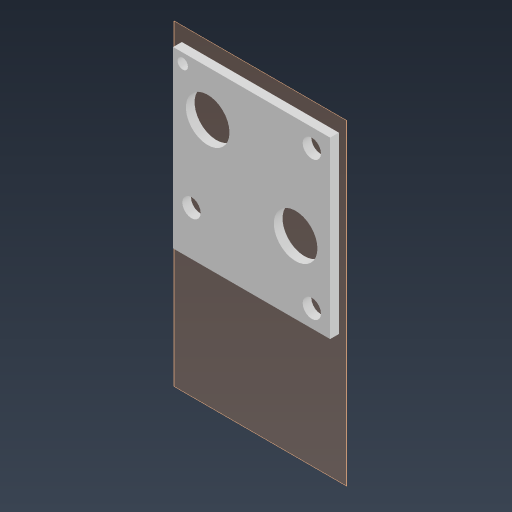
# Autodesk Inventor part: water line connector
Saved by Autodesk Inventor 2024.3 (Build 283343000, 343)
## iProperties
Created: 2024-03-20
Part Number: water line connector
Material: Generic
Document SubType Name: Modeling
Designer: mateu
Density: 1 g/cm^3
Appearance: Default
Author: mateu
Autodesk Inventor part; units mm, degrees
ref_plane "YZ Plane" through (0, 0, 0) normal (1, 0, 0) x (0, 1, 0)
ref_plane "XZ Plane" through (0, 0, 0) normal (0, 1, 0) x (-1, 0, 0)
ref_plane "Work Plane1" through (-8, -18, 2.25) normal (0, 0, 1) x (1, 0, 0)
ref_plane "Work Plane2" through (16.1776, -21.6969, -6.3588) normal (0, 0, 1) x (1, 0, 0)
sketch "Sketch6" plane through (16.1776, -21.6969, -6.3588) normal (0, 0, 1) x (1, 0, 0)
  circle A0 centre (6.9, -9.5) radius 1.2 projected
  circle A1 centre (-6.9, -6.4) radius 1.2 projected
  circle A2 centre (6.9, 6.4) radius 1.2 projected
  circle A3 centre (-7.9, 7.4) radius 0.4 projected
  line L0 (4.2, -7) -> (-1.2, -7) projected
  arc A4 (-8.5, 0.3) -> (-1.2, -7) centre (-1.2, 0.3) ccw projected
  line L1 (-8.5, 0.3) -> (-8.5, 2.7) projected
  arc A5 (-4.2, 7) -> (-8.5, 2.7) centre (-4.2, 2.7) ccw projected
  line L2 (-4.2, 7) -> (1.2, 7) projected
  arc A6 (8.5, -0.3) -> (1.2, 7) centre (1.2, -0.3) ccw projected
  line L3 (8.5, -0.3) -> (8.5, -2.7) projected
  arc A7 (4.2, -7) -> (8.5, -2.7) centre (4.2, -2.7) ccw projected
  line L4 (-4.2738, -7.5) -> (-4.2738, -24.5) projected
  line L5 (-4.2738, -7.5) -> (4.2738, -7.5) projected
  line L6 (4.2738, -24.5) -> (4.2738, -7.5) projected
  line L7 (9, -24.5) -> (4.2738, -24.5) projected
  line L8 (9, -24.5) -> (9, 8.5) projected
  line L9 (9, 8.5) -> (-9, 8.5) projected
  line L10 (-9, 8.5) -> (-9, -24.5) projected
  line L11 (-4.2738, -24.5) -> (-9, -24.5) projected
  line L12 (1.2, 6.2) -> (-4.2, 6.2) projected
  arc A8 (-4.2, 6.2) -> (-7.7, 2.7) centre (-4.2, 2.7) ccw projected
  line L13 (-7.7, 2.7) -> (-7.7, 0.3) projected
  arc A9 (-7.7, 0.3) -> (-1.2, -6.2) centre (-1.2, 0.3) ccw projected
  line L14 (-1.2, -6.2) -> (4.2, -6.2) projected
  arc A10 (4.2, -6.2) -> (7.7, -2.7) centre (4.2, -2.7) ccw projected
  line L15 (7.7, -2.7) -> (7.7, -0.3) projected
  arc A11 (7.7, -0.3) -> (1.2, 6.2) centre (1.2, -0.3) ccw projected
  line L16 (-7.2, 0.3) -> (-7.2, 2.7) projected
  arc A12 (-4.2, 5.7) -> (-7.2, 2.7) centre (-4.2, 2.7) ccw projected
  line L17 (-4.2, 5.7) -> (1.2, 5.7) projected
  arc A13 (7.2, -0.3) -> (1.2, 5.7) centre (1.2, -0.3) ccw projected
  line L18 (7.2, -0.3) -> (7.2, -2.7) projected
  arc A14 (4.2, -5.7) -> (7.2, -2.7) centre (4.2, -2.7) ccw projected
  line L19 (4.2, -5.7) -> (-1.2, -5.7) projected
  arc A15 (-7.2, 0.3) -> (-1.2, -5.7) centre (-1.2, 0.3) ccw projected
  line L20 (8.5, -0.3) -> (8.5, -2.7) projected
  arc A16 (8.5, -0.3) -> (1.2, 7) centre (1.2, -0.3) ccw projected
  line L21 (-4.2, 7) -> (1.2, 7) projected
  arc A17 (-4.2, 7) -> (-8.5, 2.7) centre (-4.2, 2.7) ccw projected
  line L22 (-8.5, 0.3) -> (-8.5, 2.7) projected
  arc A18 (-8.5, 0.3) -> (-1.2, -7) centre (-1.2, 0.3) ccw projected
  line L23 (4.2, -7) -> (-1.2, -7) projected
  arc A19 (4.2, -7) -> (8.5, -2.7) centre (4.2, -2.7) ccw projected
  arc A20 (-4.2, 6.2) -> (-7.7, 2.7) centre (-4.2, 2.7) ccw projected
  line L24 (1.2, 6.2) -> (-4.2, 6.2) projected
  arc A21 (7.7, -0.3) -> (1.2, 6.2) centre (1.2, -0.3) ccw projected
  line L25 (7.7, -2.7) -> (7.7, -0.3) projected
  arc A22 (4.2, -6.2) -> (7.7, -2.7) centre (4.2, -2.7) ccw projected
  line L26 (-1.2, -6.2) -> (4.2, -6.2) projected
  arc A23 (-7.7, 0.3) -> (-1.2, -6.2) centre (-1.2, 0.3) ccw projected
  line L27 (-7.7, 2.7) -> (-7.7, 0.3) projected
  line L28 (-1.4516, 1.7) -> (-0.5158, 1.7) projected
  arc A24 (2.07, 0.2211) -> (-0.5158, 1.7) centre (-0.5158, -1.3) ccw projected
  line L29 (2.07, 0.2211) -> (2.3135, -0.193) projected
  arc A25 (1.4516, -1.7) -> (2.3135, -0.193) centre (1.4516, -0.7) ccw projected
  line L30 (1.4516, -1.7) -> (0.5158, -1.7) projected
  arc A26 (-2.07, -0.2211) -> (0.5158, -1.7) centre (0.5158, 1.3) ccw projected
  line L31 (-2.07, -0.2211) -> (-2.3135, 0.193) projected
  arc A27 (-1.4516, 1.7) -> (-2.3135, 0.193) centre (-1.4516, 0.7) ccw projected
  arc A28 (-7.2, 0.3) -> (-1.2, -5.7) centre (-1.2, 0.3) ccw projected
  line L32 (-1.2, -5.7) -> (4.2, -5.7) projected
  arc A29 (4.2, -5.7) -> (7.2, -2.7) centre (4.2, -2.7) ccw projected
  line L33 (7.2, -2.7) -> (7.2, -0.3) projected
  arc A30 (7.2, -0.3) -> (1.2, 5.7) centre (1.2, -0.3) ccw projected
  line L34 (1.2, 5.7) -> (-4.2, 5.7) projected
  arc A31 (-4.2, 5.7) -> (-7.2, 2.7) centre (-4.2, 2.7) ccw projected
  line L35 (-7.2, 2.7) -> (-7.2, 0.3) projected
  line L36 (-9, 8.5) -> (9, 8.5)
  line L37 (9, 8.5) -> (9, -11.5)
  line L38 (9, -11.5) -> (-9, -11.5)
  line L39 (-9, -11.5) -> (-9, 8.5)
  circle A32 centre (-6.9, -6.4) radius 1.05
  circle A33 centre (6.9, -9.5) radius 1.05
  circle A34 centre (6.9, 6.4) radius 1.05
  circle A35 centre (-7.9, 7.4) radius 0.6
  circle A36 centre (-7.9, 7.4) radius 2.25
  line L40 (-4.2, 2.7) -> (4.2, -2.7)
  line L41 (-4.2, 2.7) -> (-5.0412, 3.2408)
  line L42 (4.2, -2.7) -> (5.0412, -3.2408)
  circle A37 centre (-5.0412, 3.2408) radius 2.5
  circle A38 centre (5.0412, -3.2408) radius 2.5
  point P0 (-16.1776, 21.6969)
  point P1 (-9, -11.5)
  dimension "d36" = 20
  dimension "d37" = 2.1
  dimension "d38" = 2.1
  dimension "d39" = 2.1
  dimension "d40" = 1.2
  dimension "d41" = 4.5
  dimension "d42" = 1
  dimension "d43" = 1
  dimension "d44" = 5
  dimension "d45" = 5
  constraints: 14 end point, 7 centre point, 7 coincident, 2 parallel, 1 horizontal, 1 perpendicular, 1 point on line
  measures "d36" distance of L36.end L37.end
  measures "d37" diameter of A32
  measures "d38" diameter of A33
  measures "d39" diameter of A34
  measures "d40" diameter of A35
  measures "d41" diameter of A36
  measures "d42" distance of L40.start L41.end
  measures "d43" distance of L40.end L42.end
  measures "d44" diameter of A37
  measures "d45" diameter of A38
extrude "Extrusion4" add sketch "Sketch6" along normal blind 3 contours A0 | A1 | A2 | A7 L3 A6 L2 A5 A36 L9 L8 L38 L6 L5 L4 L10 L1 A4 L0 | L0 A4 L1 A5 A36 L2 A6 L3 A7 | A36 L10 L9 A5 | A5 A36 | L4 L5 L6 L38 | A11 L15 A10 A38 L18 A13 L17 A12 A37 A8 L12 | A37 L16 A15 L19 A14 A38 A10 L14 A9 L13 A8 | A12 L17 A13 L18 A38 L40 A25 L29 A24 L28 A27 A37 | A37 L40 A27 L31 A26 L30 A25 A38 A14 L19 A15 L16 | L40 A25 L30 A26 L31 A27 | A27 L28 A24 L29 A25 L40
move faces "Move2" translate (0, 0, -2) faces at (13.0665, -31.2809, -3.3588)
body "Solid2"
